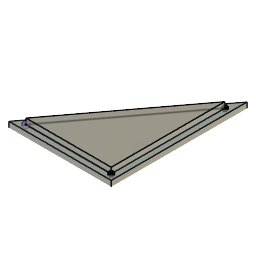
new tail v1 (Autodesk Fusion 360 design; units mm, degrees)
Autodesk Fusion 360 part; units mm, degrees
note: some values were not read from the file. Set by a fixed rule: which sketch regions a step uses.
sketch "Sketch2" plane through (0, 0, 0) normal (0, 0, 1) x (1, 0, 0)
  line L0 (29.132, 0.0089) -> (29.132, 38.6811)
  line L1 (0, 0) -> (30.132, 40.0089)
  line L2 (29.132, 2.0047) -> (8.5, 2.0047)
  line L3 (8.5, 4.0047) -> (29.132, 4.0047)
  line L4 (29.132, 4.0047) -> (29.132, 2.0047)
  line L5 (29.132, 6.0028) -> (11.5, 6.0028)
  line L6 (11.5, 8.0028) -> (29.132, 8.0028)
  line L7 (29.132, 8.0028) -> (29.132, 6.0028)
  line L8 (29.132, 10.0082) -> (14.5053, 10.0082)
  line L9 (14.5053, 12.0082) -> (29.132, 12.0082)
  line L10 (29.132, 12.0082) -> (29.132, 10.0082)
  line L11 (29.132, 13.9988) -> (17.5, 13.9988)
  line L12 (17.5, 15.9988) -> (29.132, 15.9988)
  line L13 (29.132, 15.9988) -> (29.132, 13.9988)
  line L14 (29.132, 17.997) -> (20.5, 17.997)
  line L15 (20.5, 19.997) -> (29.132, 19.997)
  line L16 (29.132, 19.997) -> (29.132, 17.997)
  line L17 (29.132, 21.9951) -> (23.5, 21.9951)
  line L18 (23.5, 23.9951) -> (29.132, 23.9951)
  line L19 (29.132, 23.9951) -> (29.132, 21.9951)
  line L20 (29.132, 25.9932) -> (26.5, 25.9932)
  line L21 (26.5, 27.9932) -> (29.132, 27.9932)
  line L22 (29.132, 27.9932) -> (29.132, 25.9932)
  line L23 (0, 0) -> (4.5764, 0.0044)
  line L24 (4.5764, 0.0044) -> (29.132, 32.609)
  line L25 (8.5, 2.0047) -> (6.0829, 2.0047)
  line L26 (6.0829, 2.0047) -> (8.5, 2.0047)
  line L27 (8.5, 4.0047) -> (6.0829, 4.0047)
  line L28 (6.0829, 4.0047) -> (6.0829, 2.0047)
  line L29 (11.5, 6.0028) -> (9.094, 6.0028)
  line L30 (9.094, 6.0028) -> (11.5, 6.0028)
  line L31 (11.5, 8.0028) -> (9.094, 8.0028)
  line L32 (9.094, 8.0028) -> (9.094, 6.0028)
  line L33 (14.5053, 10.0082) -> (12.1106, 10.0082)
  line L34 (12.1106, 10.0082) -> (12.1106, 12.0009)
  line L35 (12.1106, 12.0009) -> (14.5053, 12.0082)
  line L36 (17.5, 13.9988) -> (15.1161, 13.9988)
  line L37 (15.1161, 13.9988) -> (17.5, 13.9988)
  line L38 (17.5, 15.9988) -> (15.1161, 15.9988)
  line L39 (15.1161, 15.9988) -> (15.1161, 13.9988)
  line L40 (20.5, 17.997) -> (18.1272, 17.997)
  line L41 (18.1272, 17.997) -> (20.5, 17.997)
  line L42 (20.5, 19.997) -> (18.1272, 19.997)
  line L43 (18.1272, 19.997) -> (18.1272, 17.997)
  line L44 (23.5, 21.9951) -> (21.1383, 21.9951)
  line L45 (21.1383, 21.9951) -> (23.5, 21.9951)
  line L46 (23.5, 23.9951) -> (21.1383, 23.9951)
  line L47 (21.1383, 23.9951) -> (21.1383, 21.9951)
  line L48 (26.5, 25.9932) -> (24.1494, 25.9932)
  line L49 (24.1494, 25.9932) -> (26.5, 25.9932)
  line L50 (26.5, 27.9932) -> (24.1494, 27.9932)
  line L51 (24.1494, 27.9932) -> (24.1494, 25.9932)
  line L52 (27.158, 29.988) -> (29, 29.988)
  line L53 (29, 29.988) -> (29, 32)
  line L54 (29.132, 0.0089) -> (27.132, 0.0089)
  line L55 (27.132, 0.0089) -> (27.132, 30)
  line L56 (29.132, 30) -> (29.132, 0.0089)
  line L57 (29.132, 38.6811) -> (30.132, 40.0089)
  line L58 (0, 0) -> (30, 0)
  line L59 (30, 0) -> (30, 40)
  dimension "d9" = 2
  dimension "d15" = 30
  dimension "d16" = 40
  constraint vertical L0
  constraint coincident L1.start L23.start
  constraint horizontal L2
  constraint horizontal L3
  constraint vertical L4
  constraint coincident L0 L2.start
  constraint horizontal L5
  constraint horizontal L6
  constraint vertical L7
  constraint coincident L0 L5.start
  constraint horizontal L8
  constraint horizontal L9
  constraint vertical L10
  constraint coincident L0 L8.start
  constraint horizontal L11
  constraint horizontal L12
  constraint vertical L13
  constraint coincident L0 L11.start
  constraint horizontal L14
  constraint horizontal L15
  constraint vertical L16
  constraint coincident L0 L14.start
  constraint horizontal L17
  constraint horizontal L18
  constraint vertical L19
  constraint coincident L0 L17.start
  constraint horizontal L20
  constraint horizontal L21
  constraint vertical L22
  constraint coincident L0 L20.start
  constraint coincident L0 L24.end
  constraint parallel L1 L24
  constraint coincident L24 L25.end
  constraint horizontal L26
  constraint horizontal L27
  constraint vertical L28
  constraint coincident L24 L29.end
  constraint horizontal L30
  constraint horizontal L31
  constraint vertical L32
  constraint coincident L24 L33.end
  constraint perpendicular L33 L34
  constraint coincident L24 L36.end
  constraint horizontal L37
  constraint horizontal L38
  constraint vertical L39
  constraint coincident L24 L40.end
  constraint horizontal L41
  constraint horizontal L42
  constraint vertical L43
  constraint coincident L24 L44.end
  constraint horizontal L45
  constraint horizontal L46
  constraint vertical L47
  constraint coincident L24 L48.end
  constraint horizontal L49
  constraint horizontal L50
  constraint vertical L51
  constraint coincident L24 L52.start
  constraint horizontal L52
  constraint vertical L53
  constraint horizontal L54
  constraint vertical L55
  constraint vertical L56
  constraint coincident L0 L57.start
  constraint coincident L1 L0.end
  constraint horizontal L58
  constraint perpendicular L58 L59
  measures "d9" distance of L11.start L12.end
  measures "d15" distance of L1.start L58.end
  measures "d16" distance of L58.end L59.end
extrude "Extrude1" add sketch "Sketch2" against normal blind 2 makes body 1
extrude "Extrude2" add sketch "Sketch2" along normal blind 2 contours L0 L2 L3 L4 L55 L56 | L0 L3 L5 L55 L56 | L0 L5 L6 L7 L55 L56 | L0 L6 L8 L55 L56 | L5 L6 L24 L29 L30 L31 L55 | L0 L8 L9 L10 L55 L56 | L0 L9 L11 L55 L56 | L8 L9 L24 L33 L35 L55 | L24 L31 L32 | L0 L11 L12 L13 L55 L56 | L0 L12 L14 L55 L56 | L11 L12 L24 L36 L37 L38 L55 | L24 L34 L35 | L0 L14 L15 L16 L55 L56 | L0 L15 L17 L55 L56 | L14 L15 L24 L40 L41 L42 L55 | L24 L38 L39 | L0 L20 L21 L22 L55 L56 | L0 L17 L18 L19 L55 L56 | L0 L18 L20 L55 L56 | L20 L21 L24 L48 L49 L50 L55 | L24 L50 L51 | L17 L18 L24 L44 L45 L46 L55 | L24 L42 L43 | L24 L46 L47 bodies 1
extrude "Extrude3" add sketch "Sketch2" along normal blind 2 contours L0 L21 L24 L55 L56 bodies 1
extrude "Extrude4" add 1 faces at (30, 13.2779, -0.6667) along direction (1, 0, 0) blind 2 on bodies 1 bodies 1
extrude "Extrude5" add 1 faces at (10.6667, 0, -0.6667) along direction (0, -1, 0) blind 2 on bodies 1 bodies 1
extrude "Extrude6" add 1 faces at (10, 13.2779, -0.6667) along direction (-0.798797, 0.6016, 0) blind 2 on bodies 1 bodies 1
sketch "Sketch3" plane through (0, 0, -2) normal (0, 0, -1) x (1, 0, 0)
  line L0 (30, -39.8336) -> (32, -39.8336)
  line L1 (32, -39.8336) -> (32, 2)
  line L2 (32, 2) -> (0, 2)
  line L3 (0, 2) -> (0, 0)
  line L4 (0, 0) -> (-1.5976, -1.2032)
  line L5 (-1.5976, -1.2032) -> (28.4024, -41.0368)
  line L6 (28.4024, -41.0368) -> (30, -39.8336)
  line L7 (-1.5976, -1.2032) -> (-4.01, 2)
  line L8 (-4.01, 2) -> (0, 2)
  line L9 (28.4024, -41.0368) -> (32, -45.8136)
  line L10 (32, -45.8136) -> (32, -39.8336)
  constraint coincident L4.end L5.start
  constraint perpendicular L4 L7
  constraint coincident L2.end L3.start
  constraint perpendicular L3 L8
  constraint coincident L5.end L6.start
  constraint perpendicular L6 L9
  constraint coincident L0.end L1.start
  constraint perpendicular L0 L10
extrude "Extrude7" add sketch "Sketch3" against normal blind 2 contours L0 L6 L9 L10 | L3 L4 L7 L8 bodies 1
sketch "Sketch4" plane through (0, 0, 0) normal (0, 0, 1) x (-1, 0, 0)
  line L0 (-32, 2) -> (-32, -45.8136)
  line L1 (-32, -45.8136) -> (4.01, 2)
  line L2 (4.01, 2) -> (-32, 2)
  line L3 (-27.132, -27.9932) -> (-27.132, -29.9534)
  line L4 (-27.132, -29.9534) -> (-29.132, -32.609)
  line L5 (-29.132, -32.609) -> (-29.132, -2.0047)
  line L6 (-29.132, -2.0047) -> (-27.132, -2.0047)
  line L7 (-27.132, -2.0047) -> (-27.132, -6.0028)
  line L8 (-27.132, -6.0028) -> (-11.5, -6.0028)
  line L9 (-11.5, -6.0028) -> (-9.094, -6.0028)
  line L10 (-9.094, -6.0028) -> (-9.094, -8.0028)
  line L11 (-9.094, -8.0028) -> (-27.132, -8.0028)
  line L12 (-27.132, -8.0028) -> (-27.132, -10.0082)
  line L13 (-27.132, -10.0082) -> (-12.1106, -10.0082)
  line L14 (-12.1106, -10.0082) -> (-12.1106, -12.0009)
  line L15 (-12.1106, -12.0009) -> (-14.5053, -12.0082)
  line L16 (-14.5053, -12.0082) -> (-27.132, -12.0082)
  line L17 (-27.132, -12.0082) -> (-27.132, -13.9988)
  line L18 (-27.132, -13.9988) -> (-17.5, -13.9988)
  line L19 (-17.5, -13.9988) -> (-15.1161, -13.9988)
  line L20 (-15.1161, -13.9988) -> (-15.1161, -15.9988)
  line L21 (-15.1161, -15.9988) -> (-27.132, -15.9988)
  line L22 (-27.132, -15.9988) -> (-27.132, -17.997)
  line L23 (-27.132, -17.997) -> (-20.5, -17.997)
  line L24 (-20.5, -17.997) -> (-18.1272, -17.997)
  line L25 (-18.1272, -17.997) -> (-18.1272, -19.997)
  line L26 (-18.1272, -19.997) -> (-27.132, -19.997)
  line L27 (-27.132, -19.997) -> (-27.132, -21.9951)
  line L28 (-27.132, -21.9951) -> (-23.5, -21.9951)
  line L29 (-23.5, -21.9951) -> (-21.1383, -21.9951)
  line L30 (-21.1383, -21.9951) -> (-21.1383, -23.9951)
  line L31 (-21.1383, -23.9951) -> (-27.132, -23.9951)
  line L32 (-27.132, -23.9951) -> (-27.132, -25.9932)
  line L33 (-27.132, -25.9932) -> (-26.5, -25.9932)
  line L34 (-26.5, -25.9932) -> (-24.1494, -25.9932)
  line L35 (-24.1494, -25.9932) -> (-24.1494, -27.9932)
  line L36 (-24.1494, -27.9932) -> (-27.132, -27.9932)
  line L37 (-30, -40) -> (-30, 0)
  line L38 (-30, 0) -> (0, 0)
  line L39 (0, 0) -> (-30, -40)
  constraint perpendicular L6 L37
  constraint coincident L38.end L39.start
  constraint perpendicular L37 L38
extrude "Extrude8" add 1 faces at (28.4653, 18.2036, 2) along direction (0, 0, 1) blind 3 on bodies 1 bodies 1
extrude "Extrude9" add sketch "Sketch4" along normal blind 10 contours L0 L1 L2 bodies 1
sketch "Sketch5" plane through (0, 0, 10) normal (0, 0, 1) x (-1, 0, 0)
  line L0 (-30, 0) -> (0, 0)
  line L1 (0, 0) -> (-30, -40)
  line L2 (-30, -40) -> (-30, 0)
  line L3 (4.01, 2) -> (-32, 2)
  line L4 (-32, 2) -> (-32, -45.8136)
  line L5 (-32, -45.8136) -> (4.01, 2)
  line L6 (-30, -40) -> (-30, 0)
  line L7 (0, 0) -> (-30, -40)
  constraint coincident L1.end L2.start
  constraint coincident L0.start L2.end
  constraint coincident L0.end L1.start
extrude "Extrude10" add sketch "Sketch5" along normal blind 2 separate body contours L0 L1 L2 L6 L7 makes body 2
sketch "Sketch6" plane through (0, 0, 10) normal (0, 0, 1) x (-1, 0, 0)
  line L0 (-30, 0) -> (0, 0)
  line L1 (0, 0) -> (-30, -40)
  line L2 (-30, -40) -> (-30, 0)
  line L3 (4.01, 2) -> (-32, 2)
  line L4 (-32, 2) -> (-32, -45.8136)
  line L5 (-32, -45.8136) -> (4.01, 2)
  line L6 (0, 0) -> (-30, 0)
  line L7 (-30, -40) -> (0, 0)
  constraint coincident L0.end L1.start
  constraint coincident L0.start L2.end
  constraint coincident L1.end L2.start
